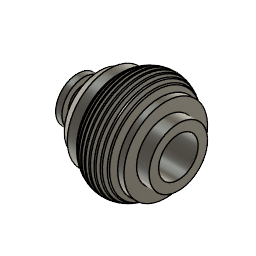
Day 8 (Autodesk Fusion 360 design; units mm, degrees)
Autodesk Fusion 360 part; units mm, degrees
sketch "Sketch1" plane through (0, 0, 0) normal (0, 1, 0) x (1, 0, 0)
  line L0 (0, -239.3605) -> (0, 80) construction
  line L1 (-170.645, -0.4139) -> (332.9489, -0.4139) construction
  line L2 (-150, -0.4139) -> (-150, -15.4139) construction
  line L3 (-150, -15.4139) -> (320.98, -15.4139) construction
  line L4 (20, -15.4139) -> (70, -15.4139)
  line L5 (20, -15.4139) -> (20, -35.4139)
  line L6 (20, -35.4139) -> (30, -35.4139)
  line L7 (30, -35.4139) -> (30, -25.4139)
  line L8 (30, -25.4139) -> (45, -25.4139)
  arc A0 (55, -35.4139) -> (45, -25.4139) centre (45, -35.4139) ccw
  line L9 (55, -35.4139) -> (55, -56.7139)
  line L10 (69.9227, -66.7794) -> (84.9227, -66.7794)
  line L11 (69.9227, -66.7794) -> (55, -56.7139)
  line L12 (69.9227, -66.7794) -> (84.9227, -66.7794) construction
  line L13 (149.9227, -66.7794) -> (159.9227, -66.7794)
  line L14 (84.9227, -66.7794) -> (84.9227, -50)
  line L15 (84.9227, -50) -> (89.9227, -50)
  line L16 (89.9227, -50) -> (89.9227, -71.7262)
  line L17 (89.9227, -71.7262) -> (91.8844, -73.2758)
  line L18 (91.8844, -73.2758) -> (91.8844, -50)
  line L19 (91.8844, -50) -> (96.8844, -50)
  line L20 (96.8844, -50) -> (96.8844, -76.4802)
  line L21 (96.8844, -76.4802) -> (99.1119, -77.6153)
  line L22 (99.1119, -77.6153) -> (99.1119, -50)
  line L23 (99.1119, -50) -> (104.1119, -50)
  line L24 (104.1119, -50) -> (104.1119, -79.6075)
  line L25 (104.1119, -79.6075) -> (106.5096, -80.3153)
  line L26 (106.5096, -80.3153) -> (106.5096, -50)
  line L27 (106.5096, -50) -> (111.5096, -50)
  line L28 (111.5096, -50) -> (111.5096, -81.3195)
  line L29 (111.5096, -81.3195) -> (113.9856, -81.6649)
  line L30 (113.9856, -81.6649) -> (113.9856, -50)
  line L31 (113.9856, -50) -> (118.9856, -50)
  line L32 (118.9856, -50) -> (118.9856, -81.7014)
  line L33 (118.9856, -81.7014) -> (121.484, -81.6101)
  line L34 (121.484, -81.6101) -> (121.484, -50)
  line L35 (121.484, -50) -> (126.484, -50)
  line L36 (126.484, -50) -> (126.484, -80.7598)
  line L37 (126.484, -80.7598) -> (128.9108, -80.1594)
  line L38 (128.9108, -80.1594) -> (128.9108, -50)
  line L39 (128.9108, -50) -> (133.9108, -50)
  line L40 (133.9108, -50) -> (133.9108, -78.4266)
  line L41 (133.9108, -78.4266) -> (136.1887, -77.3965)
  line L42 (136.1887, -77.3965) -> (136.1887, -50)
  line L43 (136.1887, -50) -> (141.1887, -50)
  line L44 (141.1887, -50) -> (141.1887, -74.5251)
  line L45 (141.1887, -74.5251) -> (143.2265, -73.0768)
  line L46 (143.2265, -73.0768) -> (143.2265, -50)
  line L47 (143.2265, -50) -> (149.9227, -50)
  line L48 (149.9227, -50) -> (149.9227, -66.7794)
  line L49 (159.9227, -66.7794) -> (159.9227, -46.7794)
  line L50 (159.9227, -46.7794) -> (179.9227, -46.7794)
  line L51 (179.9227, -46.7794) -> (179.9227, -31.7794)
  line L52 (179.9227, -31.7794) -> (70, -31.7794)
  line L53 (70, -15.4139) -> (70, -31.7794)
  line L54 (50.2219, -35.4139) -> (50.2219, -46.0639) construction
  line L55 (50.2219, -46.0639) -> (80, -46.0639) construction
  line L56 (52.4714, -46.0639) -> (52.4714, -48.5639) construction
  line L57 (52.4714, -46.0639) -> (52.4714, -43.5639) construction
  line L58 (55, -48.5639) -> (70, -48.5639)
  line L59 (55, -43.5639) -> (70, -43.5639)
  line L60 (70, -48.5639) -> (72.9773, -46.0622)
  line L61 (70, -43.5639) -> (72.9794, -46.0639)
  line L62 (70, -43.5639) -> (77.0884, -43.5639) construction
  point P0 (45, -25.4139)
  dimension "d1" = 15
  dimension "d2" = 50
  dimension "d3" = 20
  dimension "d4" = 10
  dimension "d5" = 10
  dimension "d9" = 15
  dimension "d10" = 10
  dimension "d11" = 21.3
  dimension "d15" = 15
  dimension "d16" = 146
  dimension "d17" = 18
  dimension "d18" = 65
  dimension "d19" = 10
  dimension "d25" = 5
  dimension "d26" = 2.5
  dimension "d27" = 5
  dimension "d28" = 2.5
  dimension "d29" = 5
  dimension "d30" = 2.5
  dimension "d31" = 5
  dimension "d32" = 2.5
  dimension "d33" = 5
  dimension "d34" = 2.5
  dimension "d35" = 5
  dimension "d36" = 2.5
  dimension "d37" = 5
  dimension "d38" = 2.5
  dimension "d39" = 5
  dimension "d40" = 2.5
  dimension "d43" = 20
  dimension "d44" = 20
  dimension "d45" = 15
  dimension "d46" = 2.5
  constraint vertical L0
  constraint horizontal L1
  constraint coincident L1 L2.start
  constraint perpendicular L1 L2
  constraint perpendicular L2 L3
  constraint coincident L3 L4.start
  constraint perpendicular L0 L4
  constraint perpendicular L3 L5
  constraint perpendicular L5 L6
  constraint perpendicular L1 L7
  constraint perpendicular L7 L8
  constraint coincident P0 L8
  constraint tangent L8 A0
  constraint tangent A0 L9
  constraint perpendicular L1 L9
  constraint coincident P0 L8.end
  constraint perpendicular L0 L10
  constraint horizontal L12
  constraint coincident L9.end L11.end
  constraint horizontal L13
  constraint perpendicular L10 L14
  constraint perpendicular L14 L15
  constraint perpendicular L18 L19
  constraint perpendicular L19 L20
  constraint perpendicular L22 L23
  constraint perpendicular L23 L24
  constraint perpendicular L26 L27
  constraint perpendicular L27 L28
  constraint parallel L28 L30
  constraint perpendicular L30 L31
  constraint perpendicular L31 L32
  constraint perpendicular L32 L35
  constraint parallel L36 L38
  constraint perpendicular L38 L39
  constraint perpendicular L39 L40
  constraint perpendicular L42 L43
  constraint perpendicular L47 L48
  constraint perpendicular L13 L49
  constraint perpendicular L49 L50
  constraint perpendicular L13 L51
  constraint perpendicular L51 L52
  constraint perpendicular L52 L53
  constraint parallel L9 L54
  constraint perpendicular L54 L55
  constraint coincident L55 L56.start
  constraint perpendicular L55 L56
  constraint symmetric L55 L56.start L57.start
  constraint symmetric L55 L56.end L57.end
  constraint coincident L9 L58.start
  constraint perpendicular L9 L58
  constraint coincident L9 L59.start
  constraint perpendicular L9 L59
  constraint horizontal L62
  constraint coincident L55 L61.end
  constraint coincident L61 L60.end
  measures "d1" distance of L2.start L2.end
  measures "d2" distance of L4.start L4.end
  measures "d3" distance of L4.start L5.end
  measures "d4" distance of L5.end L6.end
  measures "d5" distance of L6.end L7.end
  measures "d9" distance of L7.end P0
  measures "d10" radius of A0
  measures "d11" distance of A0.start L9.end
  measures "d15" distance of L10.start L10.end
  measures "d16" angle of L11 L12
  measures "d17" distance of L10.start L9.end
  measures "d18" distance of L10.end L13.start
  measures "d19" distance of L13.start L13.end
  measures "d25" distance of L14.end L15.end
  measures "d26" distance of L16.end L17.end
  measures "d27" distance of L18.end L19.end
  measures "d28" distance of L20.end L21.end
  measures "d29" distance of L22.end L23.end
  measures "d30" distance of L24.end L25.end
  measures "d31" distance of L26.end L27.end
  measures "d32" distance of L28.end L29.end
  measures "d33" distance of L30.end L31.end
  measures "d34" distance of L32.end L33.end
  measures "d35" distance of L34.end L35.end
  measures "d36" distance of L36.end L37.end
  measures "d37" distance of L38.end L39.end
  measures "d38" distance of L40.end L41.end
  measures "d39" distance of L42.end L43.end
  measures "d40" distance of L44.end L45.end
  measures "d43" distance of L13.end L49.end
  measures "d44" distance of L49.end L50.end
  measures "d45" distance of L50.end L51.end
  measures "d46" distance of L56.start L56.end
revolve "Revolve1" add sketch "Sketch1" angle 360 about axis through (-170.645, 0, 0.4139) along (1, 0, 0) contours L4 L5 L6 L7 L8 A0 L9 L10 L11 L13 L14 L15 L16 L17 L18 L19 L20 L21 L22 L23 L24 L25 L26 L27 L28 L29 L30 L31 L32 L33 L34 L35 L36 L37 L38 L39 L40 L41 L42 L43 L44 L45 L46 L47 L48 L49 L50 L51 L52 L53 L58 L59 L60 L61
